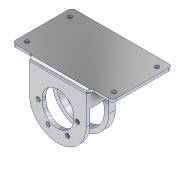
# Autodesk Inventor part: 12v DC motor mount (3D printed)
Saved by Autodesk Inventor 2022 (Build 260153000, 153)
## iProperties
Created: 2024-06-07
Part Number: 12v DC motor mount (3D printed)
Material: Generic
Document SubType Name: Sheet Metal
Designer: david
Density: 1 g/cm^3
Sheet Metal Rule: Default_mm
Appearance: Aluminum - Flat
Author: david
Autodesk Inventor part; units mm, degrees
ref_plane "YZ Plane" through (0, 0, 0) normal (1, 0, 0) x (0, 1, 0)
ref_plane "XZ Plane" through (0, 0, 0) normal (0, 1, 0) x (-1, 0, 0)
ref_plane "XY Plane" through (0, 0, 0) normal (0, 0, 1) x (1, 0, 0)
sketch "Sketch2" plane through (0, 0, 0) normal (0, 1, 0) x (-1, 0, 0)
  line L0 (22.5, 0) -> (-22.5, 0)
  line L1 (-22.5, 0) -> (-22.5, -50)
  line L2 (-22.5, -50) -> (22.5, -50)
  line L3 (22.5, -50) -> (22.5, 0)
  point P0 (0, 0)
  point P1 (0, 0)
  dimension "d4" = 50
  dimension "d5" = 45
  constraints: 8 end point, 2 coincident, 2 parallel, 1 horizontal, 1 midpoint, 1 perpendicular
  measures "d4" distance of L2.end L0.start
  measures "d5" distance between parallel lines of L1 L3
extrude "Extrusion1" add sketch "Sketch2" against normal blind 2
sketch "Sketch1" plane through (0, 0, 0) normal (0, 0, 1) x (1, 0, 0)
  line L0 (0, 0) -> (0, -25) construction
  line L1 (-22.5, 0) -> (-22.5, -25)
  line L2 (22.5, -25) -> (22.5, 0)
  arc A0 (22.5, 0) -> (-22.5, 0) centre (0, 0) ccw construction
  arc A1 (-22.5, -25) -> (22.5, -25) centre (0, -25) ccw
  circle A2 centre (0, -25) radius 18.5 construction
  line L3 (22.5, 0) -> (-22.5, 0)
  line L4 (22.5, 0) -> (22.5, -2)
  line L5 (22.5, -2) -> (-22.5, -2)
  line L6 (-22.5, -2) -> (-22.5, 0)
  line L7 (-22.5, 0) -> (22.5, 0)
  point P0 (0, -12.5)
  point P1 (0, -6.5)
  dimension "d1" = 37
  dimension "d3" = 6.5
  measures "d3" distance of L0.start point (0, -6.5)
sheet face with bend "Face1" sketch "Sketch1" thickness 2 toward (0, 0, -1) bend radius 0.5 relief straight relief width 2 relief depth 1 contours L5 L2 A1 L1
bend "Bend1"
sketch "Sketch8" plane through (0, 0, 0) normal (0, 1, 0) x (1, 0, 0)
  line L0 (-40, 2.5) -> (40, 2.5)
  line L1 (40, 2.5) -> (40, 50)
  line L2 (40, 50) -> (-40, 50)
  line L3 (-40, 50) -> (-40, 2.5)
  line L4 (-40, 2.5) -> (40, 50) construction
  line L5 (40, 2.5) -> (-40, 50) construction
  line L6 (22.5, 50) -> (-22.5, 50) projected
  line L7 (-22.5, 2.5) -> (22.5, 2.5) projected
  point P0 (0, 0)
  point P1 (0, 26.25)
  point P2 (0, 26.25)
  dimension "d50" = 80
  constraints: 12 end point, 3 midpoint, 2 collinear, 2 parallel, 1 horizontal, 1 perpendicular, 1 vertical alignment
  measures "d50" distance between parallel lines of L3 L1
extrude "Extrusion3" add sketch "Sketch8" against normal up to surface (2 mm away)
sketch "Sketch3" plane through (0, 0, 0) normal (0, 0, 1) x (1, 0, 0)
  circle A0 centre (0, -25) radius 15.5
  arc A1 (-22.5, -25) -> (22.5, -25) centre (0, -25) ccw projected
  point P0 (0, 0)
  point P1 (-15.5, -25)
  point P2 (15.5, -25)
  point P3 (-7.75, -11.5766)
  point P4 (7.75, -38.4234)
  point P5 (-7.75, -38.4234)
  point P6 (7.75, -11.5766)
  dimension "d14" = 31
  dimension "d17" = 360
  constraints: 2 horizontal alignment, 2 point on circle, 1 centre point, 1 concentric, 7 other
  measures "d14" diameter of A0
hole "Hole1" at (-15.5, -25, 0) at (15.5, -25, 0) at (7.75, -38.4234, 0) at (-7.75, -38.4234, 0) direction (0, 0, -1) diameter 3.4 end through all
sketch "Sketch4" plane through (0, 0, 0) normal (0, 1, 0) x (1, 0, 0)
  line L0 (-34.5, 43) -> (34.5, 43) construction
  line L1 (34.5, 43) -> (34.5, 9) construction
  line L2 (34.5, 9) -> (-34.5, 9) construction
  line L3 (-34.5, 9) -> (-34.5, 43) construction
  line L4 (22.5, 50) -> (-22.5, 50) construction
  point P0 (0, 0)
  point P1 (0, 43)
  point P2 (0, 50)
  dimension "d26" = 34
  dimension "d27" = 69
  dimension "d36" = 7
  constraints: 8 end point, 2 midpoint, 2 parallel, 1 horizontal, 1 perpendicular, 1 vertical alignment
  measures "d26" distance of L0.end L1.end
  measures "d27" distance of L0.start L0.end
  measures "d36" distance between parallel lines of L4 L0
hole "Hole2" at (-34.5, 0, -43) at (-34.5, 0, -9) at (34.5, 0, -43) at (34.5, 0, -9) direction (0, -1, 0) diameter 3.4 end through all
sketch "Sketch6" plane through (0, 0, 0) normal (0, 0, 1) x (1, 0, 0)
  line L0 (0, -23) -> (0, -25) construction
  line L1 (-12.5, -23) -> (-12.5, -25)
  line L2 (12.5, -25) -> (12.5, -23)
  arc A0 (12.5, -23) -> (-12.5, -23) centre (0, -23) ccw
  arc A1 (-12.5, -25) -> (12.5, -25) centre (0, -25) ccw
  arc A2 (-22.5, -25) -> (22.5, -25) centre (0, -25) ccw projected
  point P0 (0, 0)
  point P1 (0, -24)
  dimension "d45" = 25
  dimension "d46" = 2
  constraints: 8 end point, 4 point on circle, 4 tangent, 2 centre point, 1 concentric, 1 midpoint, 1 parallel, 1 vertical
  measures "d45" diameter of A1
  measures "d46" distance of L0.end L0.start
extrude "Extrusion2" cut sketch "Sketch6" against normal through all
thicken "Thicken2" operation add thickness 1 both sides no extend neighbours yes toward (0, 0, 1) faces at (-0.5022, -5.197, 0)
fillet "Fillet2" radius 3 6 edges at (-40, -1, -2.5) (-40, -1, -50) (40, -1, -2.5) (40, -1, -50) (22.5, -1, -2.5) (-22.5, -1, -2.5)
ref_plane "Work Plane1" through (0, -25, -17) normal (0, 0, 1) x (1, 0, 0)
sketch "Sketch10" plane through (0, -25, -17) normal (0, 0, 1) x (1, 0, 0)
  arc A0 (-12.5, 0) -> (12.5, 0) centre (0, 0) ccw projected
  circle A1 centre (0, 0) radius 19
  line L0 (0, 0) -> (0, 23) construction
  line L1 (22.5, 23) -> (-22.5, 23) projected
  line L2 (-22.5, 0) -> (-22.5, 23)
  line L3 (22.5, 23) -> (22.5, 0)
  arc A2 (-22.5, 0) -> (22.5, 0) centre (0, 0) ccw
  arc A3 (22.5, 23) -> (-22.5, 23) centre (0, 23) ccw construction
  arc A4 (-22.5, 0) -> (22.5, 0) centre (0, 0) ccw projected
  line L4 (37, 23) -> (-37, 23) projected
  point P0 (19.5, 23)
  point P1 (-19.5, 23)
  point P2 (0, 11.5)
  dimension "d69" = 38
  constraints: 8 end point, 4 point on circle, 4 tangent, 3 centre point, 2 midpoint, 1 coincident, 1 parallel
  measures "d69" diameter of A1
extrude "Extrusion4" add sketch "Sketch10" against normal blind 5
sketch "Sketch12" plane through (-22.5, -25, -2) normal (-1, 0, 0) x (0, 0, 1)
  line L0 (3, 22.5) -> (3, 0) projected
  line L1 (3, 11) -> (-20, 11)
  line L2 (-20, 11) -> (-34, 23)
  line L3 (-45, 23) -> (-3.5, 23) projected
  line L4 (-20, 0) -> (-20, 23) projected
  line L5 (-15, 23) -> (-15, 0) projected
  line L6 (0, 22.5) -> (0, 0) projected
  line L7 (0, 22.5) -> (0, 23)
  line L8 (0, 23) -> (-3.5, 23)
  point P0 (2, 25)
  point P1 (-15, 11)
  point P2 (0, 11)
  dimension "d72" = 12
  dimension "d73" = 14
  constraints: 8 end point, 3 point on line, 1 coincident, 1 collinear, 1 horizontal, 1 vertical
  measures "d72" distance from line of L3 L1.start
  measures "d73" distance from line of L4 point (-34, 23)
extrude "Extrusion5" add sketch "Sketch12" against normal blind 3 contours L1 L5 L3 L8 L7 L6 | L2 L3 L4
mirror "Mirror2" about plane through (0, 0, 0) normal (1, 0, 0) of "Extrusion5"
equation "\"d24\" = Thickness"
equation "\"d8\" = Thickness"
equation "\"d10\" = BendReliefWidth"
equation "\"d12\" = MinimumRemnant"
equation "\"d11\" = BendReliefDepth"
equation "\"d13\" = TransitionRadius"
equation "\"BendRadius\" = Thickness"
equation "\"BendReliefWidth\" = Thickness"
equation "\"BendReliefDepth\" = 0.5 * Thickness"
equation "\"CornerReliefSize\" = 4 * Thickness"
equation "\"MinimumRemnant\" = 2 * Thickness"
equation "\"TransitionRadius\" = BendRadius"
equation "\"JacobiRadiusSize\" = BendRadius"
equation "\"GapSize\" = Thickness"
equation "\"Thickness\" = 2"
body "Solid1"
